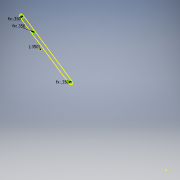
# Autodesk Inventor part: Part12
Saved by Autodesk Inventor 2016 (Build 200138000, 138)
## iProperties
Created: 2017-09-07
Part Number: Part12
Material: Generic
Document SubType Name: Modeling
Designer: student
Density: 1 g/cm^3
Appearance: Default
Author: student
Autodesk Inventor part; units mm, degrees
ref_plane "YZ Plane" through (0, 0, 0) normal (1, 0, 0) x (0, 1, 0)
ref_plane "XZ Plane" through (0, 0, 0) normal (0, 1, 0) x (-1, 0, 0)
ref_plane "XY Plane" through (0, 0, 0) normal (0, 0, 1) x (1, 0, 0)
sketch "Sketch1" plane through (0, 0, 0) normal (0, 0, 1) x (1, 0, 0)
  circle A0 centre (-377.9563, 151.9963) radius 4.445
  circle A1 centre (-272.2465, 81.6053) radius 4.445
  circle A2 centre (-409.6686, 173.1136) radius 4.445
  line L0 (-413.1881, 167.8282) -> (-275.7661, 76.3199) projected
  arc A3 (-406.1491, 178.399) -> (-413.1881, 167.8282) centre (-409.6686, 173.1136) ccw projected
  line L1 (-268.727, 86.8907) -> (-406.1491, 178.399) projected
  arc A4 (-275.7661, 76.3199) -> (-268.727, 86.8907) centre (-272.2465, 81.6053) ccw projected
  circle A5 centre (-358.9063, 119.0008) radius 4.445 construction
  point P0 (0, 0)
  dimension "d0" = 8.89
  dimension "d1" = 8.89
  dimension "d2" = 8.89
  dimension "d3" = 8.89
  constraints: 3 centre point
  measures "d0" diameter of A2
  measures "d1" diameter of A0
  measures "d2" diameter of A1
  measures "d3" diameter of A5
extrude "Extrusion1" add sketch "Sketch1" along normal blind 3.175
equation "\"d0\" = d3"
equation "\"d1\" = d3"
equation "\"d2\" = d3"
body "Solid1"
